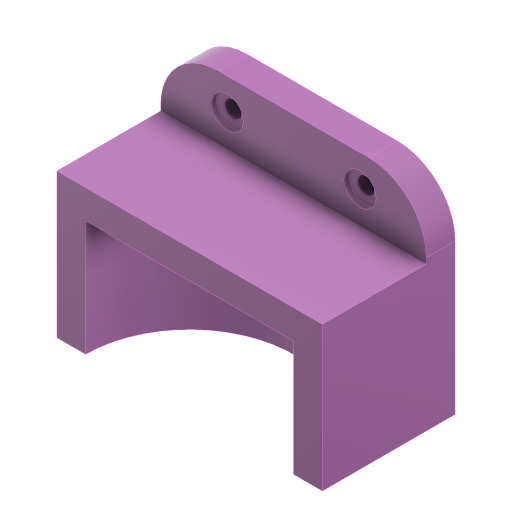
# Autodesk Inventor part: Подставка динамика
Saved by Autodesk Inventor 2023 (Build 270158000, 158)
## iProperties
Created: 2023-03-26
Part Number: Подставка динамика
Material: Типовые
Document SubType Name: Modeling
Designer: Admin
Density: 1 g/cm^3
Appearance: По умолчанию
Author: Admin
Autodesk Inventor part; units mm, degrees
ref_plane "YZ Plane" through (0, 0, 0) normal (1, 0, 0) x (0, 1, 0)
ref_plane "XZ Plane" through (0, 0, 0) normal (0, 1, 0) x (-1, 0, 0)
ref_plane "XY Plane" through (0, 0, 0) normal (0, 0, 1) x (1, 0, 0)
sketch "Эскиз1" plane through (0, 0, 0) normal (0, 0, 1) x (1, 0, 0)
  line L0 (-46, 0) -> (0, 0)
  line L1 (0, 25) -> (-46, 25)
  line L2 (-46, 25) -> (-46, 0)
  line L3 (0, 0) -> (0, 25)
  line L4 (-46, 25) -> (0, 25)
  line L5 (0, 25) -> (0, 26)
  line L6 (-10, 36) -> (-36, 36)
  circle A0 centre (-11.5, 30.5) radius 1.5
  line L7 (-11.5, 33.6177) -> (-8.8, 32.0588)
  line L8 (-8.8, 32.0588) -> (-8.8, 28.9412)
  line L9 (-8.8, 28.9412) -> (-11.5, 27.3823)
  line L10 (-11.5, 27.3823) -> (-14.2, 28.9412)
  line L11 (-14.2, 28.9412) -> (-14.2, 32.0588)
  line L12 (-14.2, 32.0588) -> (-11.5, 33.6177)
  line L13 (-14.25, 25.75) -> (-8.75, 25.75)
  line L14 (-6.75, 27.75) -> (-6.75, 33.25)
  line L15 (-8.75, 35.25) -> (-14.25, 35.25)
  line L16 (-16.25, 33.25) -> (-16.25, 27.75)
  line L17 (-16.25, 25.75) -> (-6.75, 35.25) construction
  line L18 (-6.75, 25.75) -> (-16.25, 35.25) construction
  arc A1 (-14.25, 35.25) -> (-16.25, 33.25) centre (-14.25, 33.25) ccw
  arc A2 (-8.75, 25.75) -> (-6.75, 27.75) centre (-8.75, 27.75) ccw
  arc A3 (-16.25, 27.75) -> (-14.25, 25.75) centre (-14.25, 27.75) ccw
  arc A4 (-6.75, 33.25) -> (-8.75, 35.25) centre (-8.75, 33.25) ccw
  line L19 (-37.25, 25.75) -> (-31.75, 25.75)
  line L20 (-29.75, 27.75) -> (-29.75, 33.25)
  line L21 (-31.75, 35.25) -> (-37.25, 35.25)
  line L22 (-39.25, 33.25) -> (-39.25, 27.75)
  line L23 (-39.25, 25.75) -> (-29.75, 35.25) construction
  line L24 (-29.75, 25.75) -> (-39.25, 35.25) construction
  circle A5 centre (-34.5, 30.5) radius 1.5
  line L25 (-31.8, 32.0588) -> (-31.8, 28.9412)
  line L26 (-31.8, 28.9412) -> (-34.5, 27.3823)
  line L27 (-34.5, 27.3823) -> (-37.2, 28.9412)
  line L28 (-37.2, 28.9412) -> (-37.2, 32.0588)
  line L29 (-37.2, 32.0588) -> (-34.5, 33.6177)
  line L30 (-34.5, 33.6177) -> (-31.8, 32.0588)
  line L31 (-46, 26) -> (-46, 25)
  arc A6 (-37.25, 35.25) -> (-39.25, 33.25) centre (-37.25, 33.25) ccw
  arc A7 (-29.75, 33.25) -> (-31.75, 35.25) centre (-31.75, 33.25) ccw
  arc A8 (-31.75, 25.75) -> (-29.75, 27.75) centre (-31.75, 27.75) ccw
  arc A9 (-39.25, 27.75) -> (-37.25, 25.75) centre (-37.25, 27.75) ccw
  arc A10 (0, 26) -> (-10, 36) centre (-10, 26) ccw
  arc A11 (-36, 36) -> (-46, 26) centre (-36, 26) ccw
  dimension "d0" = 25
  dimension "d1" = 5.4
  dimension "d2" = 10
  dimension "d3" = 2
  dimension "d4" = 2
  dimension "d5" = 9.5
  dimension "d6" = 3
  dimension "d7" = 4
  dimension "d8" = 4
  dimension "d9" = 9.5
  dimension "d10" = 5.4
  dimension "d11" = 4
  dimension "d12" = 10
  dimension "d13" = 2
  dimension "d14" = 10
  dimension "d15" = 46
  constraints: 65 end point, 20 point on circle, 20 tangent, 16 point on line, 12 centre point, 8 perpendicular, 7 equal radius, 5 parallel, 4 coincident, 4 midpoint, 3 horizontal, 3 vertical, 1 collinear, 26 other
  measures "d0" distance of L0.start L1.end
  measures "d1" distance between parallel lines of L11 L8
  measures "d2" distance edge to line of A0 L5
  measures "d3" radius of A1
  measures "d4" radius of A2
  measures "d5" distance between parallel lines of L13 L15
  measures "d6" diameter of A0
  measures "d7" distance edge to line of A0 L6
  measures "d8" distance edge to line of A0 L1
  measures "d9" distance between parallel lines of L22 L20
  measures "d10" distance between parallel lines of L27 L30
  measures "d11" distance edge to line of A5 L6
  measures "d12" distance edge to line of A5 L31
  measures "d13" radius of A6
  measures "d14" radius of A10
  measures "d15" distance of L0.start L0.end
extrude "Выдавливание1" add sketch "Эскиз1" along normal blind 23 contours L2 L1 L3 L0
extrude "Выдавливание2" add sketch "Эскиз1" along normal blind 5 contours L31 A11 L6 A10 L5 L1 | L7 L8 L9 L10 L11 L12 | A3 L16 A1 L15 A4 L14 A2 L13 | A9 L22 A6 L21 A7 L20 A8 L19 | L25 L26 L27 L28 L29 L30
sketch "Эскиз2" plane through (0, 0, 5) normal (0, 0, 1) x (1, 0, 0)
  circle A0 centre (-34.5, 30.5) radius 2.8
  circle A1 centre (-11.5, 30.5) radius 1.5 projected
  circle A2 centre (-11.5, 30.5) radius 2.8
  point P0 (0, 0)
  constraints: 2 centre point, 2 coincident, 1 equal radius, 1 other
extrude "Выдавливание3" cut sketch "Эскиз2" against normal blind 1 contours A0 | A1 | A2
sketch "Эскиз3" plane through (-46, 0, 0) normal (0, -1, 0) x (1, 0, 0)
  line L0 (0, 23) -> (46, 23) projected
  line L1 (46, 23) -> (0, 23) projected
  circle A0 centre (23, 23) radius 18
  point P0 (46, 0)
  dimension "d23" = 36
  constraints: 1 centre point, 1 midpoint
  measures "d23" diameter of A0
extrude "Выдавливание4" cut sketch "Эскиз3" against normal blind 20
